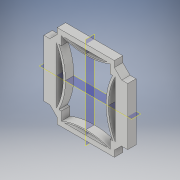
# Autodesk Inventor part: 20_Cube_Insert_Lens_Cylindrical_v3
Saved by Autodesk Inventor 2019 (Build 230136000, 136)
## iProperties
Created: 2019-07-24
Part Number: 20_Cube_Insert_Lens_Cylindrical_v3
Material: Generic
Document SubType Name: Modeling
Designer: marsikovabarbora
Density: 1 g/cm^3
Appearance: Default
Author: marsikovabarbora
Autodesk Inventor part; units mm, degrees
ref_plane "YZ Plane" through (0, 0, 0) normal (1, 0, 0) x (0, 1, 0)
ref_plane "XZ Plane" through (0, 0, 0) normal (0, 1, 0) x (-1, 0, 0)
ref_plane "XY Plane" through (0, 0, 0) normal (0, 0, 1) x (1, 0, 0)
sketch "Sketch1" plane through (0, 0, 0) normal (0, 0, 1) x (1, 0, 0)
  line L0 (21.5871, 13.6345) -> (17.0871, 18.1345) projected
  line L1 (17.0871, 18.1345) -> (-16.7129, 18.1345) projected
  line L2 (-16.7129, 18.1345) -> (-21.2129, 13.6345) projected
  line L3 (-21.0966, 13.6345) -> (-21.0966, -20.1655) projected
  line L4 (21.4709, -20.1655) -> (21.4709, 13.6345) projected
  line L5 (21.4709, -20.1655) -> (17.0871, -24.4078) projected
  line L6 (-16.7129, -24.4078) -> (17.0871, -24.4078) projected
  line L7 (-16.7129, -24.4078) -> (-21.0966, -20.1655) projected
  line L8 (-24.7129, -28.1655) -> (-24.7129, 13.6345) construction
  line L9 (25.0871, -28.1655) -> (-24.7129, -28.1655) construction
  line L10 (25.0871, -28.1655) -> (25.0871, 13.6345) construction
  line L11 (17.0871, 21.6345) -> (-16.7129, 21.6345) construction
  line L12 (-21.0552, -20.0655) -> (-16.6129, -24.5078)
  line L13 (-16.6129, -24.5078) -> (-16.6129, -28.1655)
  line L14 (-16.6129, -28.1655) -> (17.0871, -28.1655)
  line L15 (25.0871, -20.0655) -> (21.4295, -20.0655)
  line L16 (25.0871, 13.5345) -> (25.0871, -20.0655)
  line L17 (21.4295, 13.5345) -> (25.0871, 13.5345)
  line L18 (21.4295, 13.5345) -> (16.9871, 17.9768)
  line L19 (16.9871, 17.9768) -> (16.9871, 21.6345)
  line L20 (16.9871, 21.6345) -> (-16.6129, 21.6345)
  line L21 (-16.6129, 21.6345) -> (-16.6129, 17.9768)
  line L22 (-16.6129, 17.9768) -> (-21.0552, 13.5345)
  line L23 (-24.7129, 13.5345) -> (-21.0552, 13.5345)
  line L24 (-24.7129, -20.0655) -> (-24.7129, 13.5345)
  line L25 (-21.0552, -20.0655) -> (-24.7129, -20.0655)
  line L26 (-12.3129, -23.2655) -> (12.6871, -23.2655) projected
  line L27 (12.6871, -23.2655) -> (12.6871, 16.7345) projected
  line L28 (-12.3129, 16.7345) -> (12.6871, 16.7345) projected
  line L29 (-12.3129, -23.2655) -> (-12.3129, 16.7345) projected
  line L30 (14.6871, -25.2655) -> (-14.3129, -25.2655) construction
  line L31 (-14.3129, -25.2655) -> (-14.3129, 18.7345) construction
  line L32 (-14.3129, 18.7345) -> (14.6871, 18.7345) construction
  line L33 (14.6871, 18.7345) -> (14.6871, -25.2655) construction
  line L34 (-17.3129, 21.7345) -> (17.6871, 21.7345) construction
  line L35 (17.6871, 21.7345) -> (17.6871, -28.2655) construction
  line L36 (17.6871, -28.2655) -> (-17.3129, -28.2655) construction
  line L37 (-17.3129, -28.2655) -> (-17.3129, 21.7345) construction
  line L38 (-14.3129, -23.2655) -> (-14.3129, -25.2655)
  line L39 (-14.3129, -25.2655) -> (14.6871, -25.2655)
  line L40 (14.6871, -25.2655) -> (14.6871, -20.0655)
  line L41 (14.6871, -20.0655) -> (17.6871, -20.0655)
  line L42 (17.6871, -20.0655) -> (17.6871, 13.5345)
  line L43 (17.6871, 13.5345) -> (14.6871, 13.5345)
  line L44 (14.6871, 13.5345) -> (14.6871, 18.7345)
  line L45 (14.6871, 18.7345) -> (-14.3129, 18.7345)
  line L46 (-14.3129, 18.7345) -> (-14.3129, 13.5345)
  line L47 (-14.3129, 13.5345) -> (-17.3129, 13.5345)
  line L48 (-17.3129, 13.5345) -> (-17.3129, -20.0655)
  line L49 (-17.3129, -20.0655) -> (-14.3129, -20.0655)
  line L50 (-14.3129, -20.0655) -> (-14.3129, -23.2655)
  line L51 (-16.6129, -28.1655) -> (17.0871, -28.1655)
  line L52 (16.9871, -28.1655) -> (16.9871, -24.3509)
  line L53 (16.9871, -24.3509) -> (21.2726, -20.0655)
  line L54 (21.2726, -20.0655) -> (21.4295, -20.0655)
  point P0 (14.2, -44.8454)
  point P1 (16.9871, 19.8057)
  dimension "d74" = 2
  dimension "d75" = 5
  dimension "d76" = 135
  constraints: 78 end point, 15 point on line, 7 horizontal, 5 vertical, 4 perpendicular, 3 collinear, 1 midpoint, 10 other
  measures "d74" distance between parallel lines of L26 L30
  measures "d75" distance between parallel lines of L29 L37
  measures "d76" angle of L52 L53
extrude "Extrusion1" add sketch "Sketch1" along normal blind 5 contours L19 L18 L17 L4 L15 L54 L53 L52 L6 L40 L41 L42 L43 L44 L1 | L1 L44 L45 L46 L21 L20 L19 | L46 L47 L48 L49 L50 L38 L6 L12 L25 L3 L23 L22 L21 L1 | L17 L16 L15 L4 | L3 L25 L24 L23 | L6 L52 L14 L13 L12 L38 L39 L40
sketch "Sketch5" plane through (0, 0, 0) normal (0, 0, -1) x (-1, 0, 0)
  line L0 (12.3129, -23.2655) -> (-12.6871, -23.2655) construction
  line L1 (-12.6871, -23.2655) -> (-12.6871, 16.7345) construction
  line L2 (12.3129, 16.7345) -> (-12.6871, 16.7345) construction
  line L3 (12.3129, -23.2655) -> (12.3129, 16.7345) construction
  line L4 (-14.6871, -25.2655) -> (14.3129, -25.2655) construction
  arc A0 (14.3129, -25.2655) -> (-0.1871, -22.4693) centre (0.3594, -58.629) ccw
  arc A1 (12.3827, -25.2655) -> (-0.1871, -23.1694) centre (0.3594, -58.629) ccw
  line L5 (-0.1871, -22.4693) -> (-0.1871, -23.1694)
  line L6 (14.3129, -20.0655) -> (14.3129, -25.2655) projected
  line L7 (14.3129, -25.2655) -> (12.3827, -25.2655)
  point P0 (0, 0)
  dimension "d79" = 0.7
  constraints: 4 end point, 4 point on circle, 2 centre point, 1 coincident, 1 point on line, 1 vertical
  measures "d79" radial gap between concentric circles of A1 A0
extrude "Extrusion4" add sketch "Sketch5" against normal up to surface (5 mm away)
mirror "Mirror1" about plane through (0.1871, -23.1694, 0) normal (1, 0, 0) of "Extrusion4"
ref_plane "Work Plane1" through (0.1871, -20.0655, 0) normal (-1, 0, 0) x (0, 0, 1)
ref_plane "Work Plane2" through (-16.6129, -3.2655, 0) normal (0, -1, 0) x (1, 0, 0)
mirror "Mirror2" about plane through (-16.6129, -3.2655, 0) normal (0, -1, 0) of "Extrusion4", "Mirror1"
sketch "Sketch6" plane through (0, 0, 0) normal (0, 0, -1) x (-1, 0, 0)
  spline S0 degree 3 poles (1.425, -3.2655) (1.425, -3.4679) (1.3845, -3.6839) (1.22, -4.081) (1.0959, -4.2623) (0.8097, -4.5486) (0.6284, -4.6726) (0.2312, -4.8371) (0.0153, -4.8776) (-0.3896, -4.8776) (-0.6055, -4.8371) (-1.0027, -4.6726) (-1.1839, -4.5486) (-1.4702, -4.2623) (-1.5943, -4.081) (-1.7588, -3.6839) (-1.7992, -3.4679) (-1.7992, -3.0631) (-1.7588, -2.8471) (-1.5943, -2.45) (-1.4702, -2.2687) (-1.1839, -1.9824) (-1.0027, -1.8584) (-0.6055, -1.6939) (-0.3896, -1.6534) (0.0153, -1.6534) (0.2312, -1.6939) (0.6284, -1.8584) (0.8097, -1.9824) (1.0959, -2.2687) (1.22, -2.45) (1.3845, -2.8471) (1.425, -3.0631) (1.425, -3.2655) knots 0 0 0 0 0.060733 0.060733 0.121465 0.121465 0.182198 0.182198 0.24293 0.24293 0.303663 0.303663 0.364395 0.364395 0.425128 0.425128 0.48586 0.48586 0.546593 0.546593 0.607326 0.607326 0.668058 0.668058 0.728791 0.728791 0.789523 0.789523 0.850256 0.850256 0.910988 0.910988 0.971721 0.971721 0.971721 0.971721 projected
  line L0 (17.3129, 13.5345) -> (17.3129, -20.0655) projected
  arc A0 (13.2973, -3.2655) -> (17.3129, -20.0655) centre (48.9305, -3.6282) ccw
  line L1 (17.3129, -20.0655) -> (14.3129, -20.0655) projected
  arc A1 (11.9598, -3.2655) -> (15.8129, -20.0655) centre (48.9305, -3.6282) ccw
  line L2 (11.9598, -3.2655) -> (13.2973, -3.2655)
  line L3 (15.8129, -20.0655) -> (17.3129, -20.0655)
  point P0 (0, 0)
  point P1 (1.425, -3.2655)
  constraints: 4 end point, 4 point on circle, 2 centre point, 1 coincident, 1 horizontal, 1 midpoint
extrude "Extrusion5" add sketch "Sketch6" against normal up to surface (5 mm away) contours A0 L1 A1 L2
mirror "Mirror3" about plane through (-11.9598, -3.2655, 0) normal (0, 1, 0) of "Extrusion5"
mirror "Mirror4" about plane through (0.1871, -20.0655, 0) normal (-1, 0, 0) of "Extrusion5", "Mirror3"
sketch "Skizze7" plane through (0, 0, 5) normal (0, 0, 1) x (1, 0, 0)
  arc A0 (12.3341, -3.2655) -> (16.1871, -20.0655) centre (49.3047, -3.6282) ccw construction
  line L0 (16.1871, -20.0655) -> (14.6871, -20.0655) projected
  line L1 (14.6871, -20.0655) -> (14.6871, -25.2655) projected
  arc A1 (14.6871, -25.2655) -> (0.1871, -22.4693) centre (0.7336, -58.629) ccw construction
  arc A2 (0.1871, -22.4693) -> (-14.3129, -25.2655) centre (-0.3594, -58.629) ccw construction
  line L2 (-14.3129, -25.2655) -> (-14.3129, -20.0655) construction
  line L3 (-14.3129, -20.0655) -> (-15.8129, -20.0655) construction
  arc A3 (-15.8129, -20.0655) -> (-11.9598, -3.2655) centre (-48.9305, -3.6282) ccw construction
  arc A4 (-11.9598, -3.2655) -> (-15.8129, 13.5345) centre (-48.9305, -2.9028) ccw construction
  line L4 (-15.8129, 13.5345) -> (-14.3129, 13.5345) construction
  line L5 (-14.3129, 13.5345) -> (-14.3129, 18.7345) construction
  arc A5 (-14.3129, 18.7345) -> (0.1871, 15.9383) centre (-0.3594, 52.098) ccw construction
  arc A6 (0.1871, 15.9383) -> (14.6871, 18.7345) centre (0.7336, 52.098) ccw construction
  line L6 (14.6871, 18.7345) -> (14.6871, 13.5345) construction
  line L7 (14.6871, 13.5345) -> (16.1871, 13.5345) construction
  arc A7 (16.1871, 13.5345) -> (12.3341, -3.2655) centre (49.3047, -2.9028) ccw construction
  arc A8 (-17.3129, -20.0655) -> (-13.2973, -3.2655) centre (-48.9305, -3.6282) ccw construction
  line L8 (-17.3129, -20.0655) -> (-17.3129, 13.5345) construction
  arc A9 (-13.2973, -3.2655) -> (-17.3129, 13.5345) centre (-48.9305, -2.9028) ccw construction
  arc A10 (17.6871, 13.5345) -> (13.6715, -3.2655) centre (49.3047, -2.9028) ccw construction
  line L9 (17.6871, 13.5345) -> (17.6871, -20.0655) construction
  arc A11 (13.6715, -3.2655) -> (17.6871, -20.0655) centre (49.3047, -3.6282) ccw construction
  line L10 (12.757, -25.2655) -> (-12.3827, -25.2655) construction
  arc A12 (0.1871, -23.1694) -> (-12.3827, -25.2655) centre (-0.3594, -58.629) ccw construction
  arc A13 (12.757, -25.2655) -> (0.1871, -23.1694) centre (0.7336, -58.629) ccw construction
  arc A14 (0.1871, 16.6384) -> (12.757, 18.7345) centre (0.7336, 52.098) ccw construction
  arc A15 (-12.3827, 18.7345) -> (0.1871, 16.6384) centre (-0.3594, 52.098) ccw construction
  line L11 (-12.3827, 18.7345) -> (12.757, 18.7345) construction
  line L12 (-21.0552, -20.0655) -> (-16.6129, -24.5078) projected
  line L13 (-16.6129, -24.5078) -> (-16.6129, -28.1655) projected
  line L14 (-16.6129, -28.1655) -> (16.9871, -28.1655) construction
  line L15 (16.9871, -28.1655) -> (16.9871, -24.3509) projected
  line L16 (16.9871, -24.3509) -> (21.2726, -20.0655) projected
  line L17 (21.2726, -20.0655) -> (25.0871, -20.0655) projected
  line L18 (25.0871, -20.0655) -> (25.0871, 13.5345) construction
  line L19 (25.0871, 13.5345) -> (21.4295, 13.5345) projected
  line L20 (21.4295, 13.5345) -> (16.9871, 17.9768) projected
  line L21 (16.9871, 17.9768) -> (16.9871, 21.6345) projected
  line L22 (16.9871, 21.6345) -> (-16.6129, 21.6345) construction
  line L23 (-16.6129, 21.6345) -> (-16.6129, 17.9768) projected
  line L24 (-16.6129, 17.9768) -> (-21.0552, 13.5345) projected
  line L25 (-21.0552, 13.5345) -> (-24.7129, 13.5345) projected
  line L26 (-24.7129, 13.5345) -> (-24.7129, -20.0655) construction
  line L27 (-24.7129, -20.0655) -> (-21.0552, -20.0655) projected
  line L28 (-16.8129, 21.8345) -> (17.1871, 21.8345) construction
  line L29 (17.1871, 21.8345) -> (17.1871, 18.0597)
  line L30 (17.1871, 18.0597) -> (21.5123, 13.7345)
  line L31 (21.5123, 13.7345) -> (25.2871, 13.7345)
  line L32 (25.2871, 13.7345) -> (25.2871, -20.2655) construction
  line L33 (25.2871, -20.2655) -> (21.3554, -20.2655)
  line L34 (21.3554, -20.2655) -> (17.1871, -24.4338)
  line L35 (17.1871, -24.4338) -> (17.1871, -28.3655)
  line L36 (17.1871, -28.3655) -> (-16.8129, -28.3655) construction
  line L37 (-16.8129, -28.3655) -> (-16.8129, -24.5907)
  line L38 (-16.8129, -24.5907) -> (-21.1381, -20.2655)
  line L39 (-21.1381, -20.2655) -> (-24.9129, -20.2655)
  line L40 (-24.9129, -20.2655) -> (-24.9129, 13.7345) construction
  line L41 (-24.9129, 13.7345) -> (-21.1381, 13.7345)
  line L42 (-21.1381, 13.7345) -> (-16.8129, 18.0597)
  line L43 (-16.8129, 18.0597) -> (-16.8129, 21.8345)
  line L44 (-21.0552, 13.5345) -> (-24.7129, 13.5345) projected
  line L45 (-24.7129, 13.5345) -> (-24.7129, 13.7345)
  line L46 (-16.6129, 21.6345) -> (-16.8129, 21.6345)
  line L47 (16.9871, 17.9768) -> (16.9871, 21.6345) projected
  line L48 (16.9871, 21.6345) -> (17.1871, 21.6345)
  line L49 (25.0871, -20.0655) -> (25.0871, 13.5345) projected
  line L50 (25.0871, 13.5345) -> (25.0871, 13.7345)
  line L51 (25.0871, -20.0655) -> (25.0871, -20.2655)
  line L52 (-16.6129, -28.1655) -> (16.9871, -28.1655) projected
  line L53 (16.9871, -28.1655) -> (17.1871, -28.1655)
  line L54 (-16.6129, -28.1655) -> (-16.8129, -28.1655)
  line L55 (-24.7129, -20.0655) -> (-24.7129, -20.2655)
  point P0 (0, 0)
  dimension "d83" = 0.2
  constraints: 48 end point, 14 point on line, 2 perpendicular, 15 other
  measures "d83" distance between parallel lines of L22 L28
extrude "IM_offset" add sketch "Skizze7" against normal up to surface (5 mm away)
body "Solid1"
